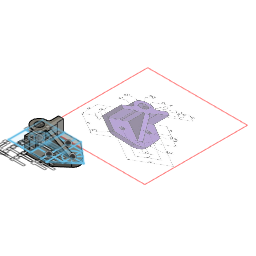
A3 v1 (Autodesk Fusion 360 design; units mm, degrees)
Autodesk Fusion 360 part; units mm, degrees
note: some values were not read from the file. Set by a fixed rule: which sketch regions a step uses.
sketch "Sketch1" plane through (0, 0, 0) normal (0, 1, 0) x (1, 0, 0)
  line L0 (-93.5789, -91) -> (-48.797, -91)
  line L1 (-48.797, -91) -> (-48.797, -179)
  line L2 (-48.797, -179) -> (-93.5789, -179)
  line L3 (-93.5789, -179) -> (-93.5789, -91)
  line L4 (-48.797, -179) -> (2.6553, -135)
  line L5 (2.6553, -135) -> (-48.797, -91)
  line L6 (-93.5789, -91) -> (-148.2679, -91)
  line L7 (-148.2679, -91) -> (-148.2679, -179)
  line L8 (-148.2679, -179) -> (-93.5789, -179)
  line L9 (2.6553, -135) -> (-148.2679, -135)
  line L10 (-90.5789, -91) -> (-90.5789, -179)
  line L11 (-26.5789, -110) -> (-26.5789, -160)
  line L12 (-26.5789, -130) -> (-90.5789, -130)
  line L13 (-26.5789, -140) -> (-90.5789, -140)
  line L14 (-26.5789, -110) -> (-90.5789, -110)
  line L15 (-26.5789, -160) -> (-90.5789, -160)
  line L16 (-62.5789, -91) -> (-62.5789, -179)
  circle A0 centre (-62.5789, -110) radius 5
  circle A1 centre (-62.5789, -160) radius 5
  line L17 (-106.5789, -91) -> (-106.5789, -179)
  line L18 (-112.5789, -91) -> (-112.5789, -179)
  line L19 (-86.5789, -140) -> (-86.5789, -130)
  circle A2 centre (-112.5789, -135) radius 9.5
  circle A3 centre (-112.5789, -135) radius 19
  line L20 (-26.5789, -135) -> (-14.2304, -120.56)
  line L21 (-26.5789, -135) -> (-14.2304, -149.44)
  circle A4 centre (-26.5789, -135) radius 19
  line L22 (-90.5789, -160) -> (-93.5789, -160)
  line L23 (-90.5789, -130) -> (-93.5789, -130)
  line L24 (-90.5789, -110) -> (-93.5789, -110)
  line L25 (-90.5789, -140) -> (-93.5789, -140)
  dimension "d1" = 3
  dimension "d2" = 5
  dimension "d3" = 10
  dimension "d4" = 50
  dimension "d7" = 88
  dimension "d8" = 67
  dimension "d10" = 31
  dimension "d11" = 36
  dimension "d12" = 10
  dimension "d13" = 10
  dimension "d16" = 13
  dimension "d17" = 19
  dimension "d18" = 20
  dimension "d19" = 19
  dimension "d20" = 38
  dimension "d22" = 19
  dimension "d23" = 19
  dimension "d24" = 13.782
  constraint horizontal L0
  constraint vertical L1
  constraint horizontal L2
  constraint vertical L3
  constraint perpendicular L3 L6
  constraint perpendicular L6 L7
  constraint perpendicular L7 L8
  constraint equal L4 L5
  constraint midpoint L7 L9.end
  constraint coincident L0 L10.start
  constraint coincident L2 L10.end
  constraint perpendicular L2 L10
  constraint coincident L5 L11.start
  constraint coincident L4 L11.end
  constraint perpendicular L9 L11
  constraint coincident L11 L12.start
  constraint coincident L10 L12.end
  constraint perpendicular L10 L12
  constraint coincident L11 L13.start
  constraint coincident L10 L13.end
  constraint perpendicular L10 L13
  constraint coincident L10 L14.end
  constraint perpendicular L10 L14
  constraint coincident L10 L15.end
  constraint perpendicular L10 L15
  constraint coincident L0 L16.start
  constraint coincident L2 L16.end
  constraint perpendicular L2 L16
  constraint coincident L14 A0.centre
  constraint coincident L16 A0.centre
  constraint coincident L15 A1.centre
  constraint coincident L16 A1.centre
  constraint coincident L6 L17.start
  constraint coincident L8 L17.end
  constraint perpendicular L8 L17
  constraint coincident L6 L18.start
  constraint coincident L8 L18.end
  constraint perpendicular L8 L18
  constraint coincident L13 L19.start
  constraint coincident L12 L19.end
  constraint perpendicular L12 L19
  constraint midpoint L18 A2.centre
  constraint concentric A2 A3
  constraint midpoint L11 L20.start
  constraint coincident L5 L20.end
  constraint perpendicular L5 L20
  constraint coincident L4 L21.end
  constraint perpendicular L4 L21
  constraint coincident L20.start L21.start
  constraint coincident L20.end A4
  constraint coincident L3 L22.end
  constraint perpendicular L3 L22
  constraint coincident L3 L23.end
  constraint perpendicular L3 L23
  constraint coincident L3 L24.end
  constraint perpendicular L3 L24
  constraint coincident L3 L25.end
  constraint perpendicular L3 L25
  measures "d1" distance of L3 L10
  measures "d2" distance of L9 L12
  measures "d3" distance of L12 L13
  measures "d4" distance of L14 L15
  measures "d7" distance of L0 L2
  measures "d8" distance of L3 L11
  measures "d10" distance of L3 L16
  measures "d11" distance of L11 L16
  measures "d12" diameter of A0
  measures "d13" diameter of A1
  measures "d16" distance of L3 L17
  measures "d17" distance of L3 L18
  measures "d18" distance of L17 L19
  measures "d19" diameter of A2
  measures "d20" diameter of A3
  measures "d22" distance of L20.start L20.end
  measures "d23" distance of L20.start L21.end
  measures "d24" distance of L1 L16
extrude "Extrude1" add sketch "Sketch1" against normal blind 10 contours L0 L3 L10 L24 | L3 L6 L17 A3 | L0 L10 L14 L16 A0 | L3 L10 L23 L24 | L0 L1 L14 L16 A0 | L10 L12 L14 L16 A0 | L3 L9 L10 L23 | L9 L17 A2 A3 | L17 L18 A2 A3 | L1 L5 L14 | L9 L10 L12 L19 | L3 L9 L10 L25 | L9 L17 A2 A3 | L3 L8 L17 A3 | L9 L18 A2 A3 | L1 L11 L12 L14 A4 | L1 L12 L14 L16 A0 | L5 L11 A4 | L9 L10 L13 L19 | L9 L12 L16 L19 | L3 L10 L22 L25 | L17 L18 A2 A3 | L9 L18 A2 A3 | L1 L9 L12 A4 | L1 L9 L12 L16 | L9 L20 A4 | L11 L20 A4 | L11 L12 A4 | L9 L13 L16 L19 | L10 L13 L15 L16 A1 | L2 L3 L10 L22 | L1 L9 L13 A4 | L1 L9 L13 L16 | L9 L11 L12 A4 | L9 L11 L13 A4 | L11 L21 A4 | L9 L21 A4 | L2 L10 L15 L16 A1 | L1 L11 L13 L15 A4 | L1 L13 L15 L16 A1 | L4 L11 A4 | L11 L13 A4 | L1 L4 L15 | L1 L2 L15 L16 A1 makes body 1
extrude "Extrude2" add sketch "Sketch1" along normal blind 30 contours L3 L6 L17 A3 | L3 L10 L23 L24 | L3 L9 L10 L23 | L9 L17 A2 A3 | L17 L18 A2 A3 | L9 L10 L12 L19 | L3 L9 L10 L25 | L9 L17 A2 A3 | L3 L8 L17 A3 | L9 L18 A2 A3 | L9 L10 L13 L19 | L3 L10 L22 L25 | L17 L18 A2 A3 | L9 L18 A2 A3 bodies 1
extrude "Extrude3" add sketch "Sketch1" along normal blind 30 separate body contours L9 L12 L16 L19 | L1 L9 L12 A4 | L1 L9 L12 L16 | L9 L13 L16 L19 | L1 L9 L13 A4 | L1 L9 L13 L16 | L9 L11 L12 A4 | L9 L11 L13 A4 makes body 2
draft "Draft1" angle -26.5 neutral plane through (-86.5789, 0, 135) pull (-1, 0, 0) 1 faces at (-70.5789, 30, 135) on bodies 2
combine "Combine1" operation add target body 2 tool bodies 1
fillet "Fillet1" radius 13 1 edges at (-48.797, -5, 179) on bodies 2
fillet "Fillet2" radius 13 1 edges at (-48.797, -5, 91) on bodies 2
fillet "Fillet3" radius 3 1 edges at (-93.5789, 15, 160) on bodies 2
fillet "Fillet4" radius 3 1 edges at (-93.5789, 15, 110) on bodies 2
fillet "Fillet5" radius 6 1 edges at (-106.5789, 10, 153.0278) on bodies 2
fillet "Fillet6" radius 6 1 edges at (-106.5789, 10, 116.9722) on bodies 2
named bodies: "A3"
